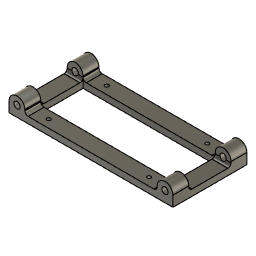
Pojezd - X v19 (Autodesk Fusion 360 design; units mm, degrees)
Autodesk Fusion 360 part; units mm, degrees
note: some values were not read from the file. Chosen so that the rebuilt part matches the saved one: which bodies a step acts on.
sketch "Sketch2" plane through (0, 0, 0) normal (0, 1, 0) x (1, 0, 0)
  circle A0 centre (0, -10) radius 3
  line L0 (147.5, -10) -> (147.5, 0)
  line L1 (147.5, 0) -> (-7.5, 0)
  line L2 (-7.5, 0) -> (-7.5, -10)
  arc A1 (-7.5, -10) -> (7.5, -10) centre (0, -10) ccw
  line L3 (7.5, -10) -> (7.5, -9)
  arc A2 (10.5, -6) -> (7.5, -9) centre (10.5, -9) ccw
  line L4 (70, 35) -> (70, -50) construction
  arc A3 (132.5, -10) -> (147.5, -10) centre (140, -10) ccw
  circle A4 centre (140, -10) radius 3
  line L5 (132.5, -10) -> (132.5, -9)
  arc A5 (132.5, -9) -> (129.5, -6) centre (129.5, -9) ccw
  line L6 (10.5, -6) -> (129.5, -6)
  dimension "d11" = 10
  dimension "d13" = 15
  dimension "d14" = 6
  dimension "d16" = 155
  dimension "d24" = 3
  dimension "d53" = 7.5
  dimension "d54" = 77.5
  dimension "d55" = 140
  dimension "d56" = 6
  dimension "d117" = 4
  constraint concentric A0 A1
  constraint vertical L0
  constraint horizontal L1
  constraint vertical L2
  constraint horizontal L6
  constraint vertical L3
  constraint tangent L3 A2
  constraint tangent A2 L6
  constraint perpendicular L4 L6
  constraint symmetric A0 L4 A4
  constraint symmetric A1 L4 A3
  constraint symmetric L2.end L4 L0.start
  constraint symmetric A1.end L4 A3.start
  constraint symmetric L3.end L4 L5.end
  constraint symmetric A2.start L4 A5.end
  constraint symmetric A2 L4 A5
  measures "d11" vertical distance of origin A0.centre
  measures "d13" diameter of A1
  measures "d14" diameter of A0
  measures "d16" distance of L0.end L1.end
  measures "d24" radius of A2
  measures "d53" distance of origin L1.end
  measures "d54" horizontal distance of L1.end L4.start
  measures "d55" distance of A0.centre A3.centre
  measures "d56" distance of L1 L6
  measures "d117" vertical distance of A0.centre A2.start
extrude "Extrude9" add sketch "Sketch2" along normal blind 70 makes body 1
sketch "Sketch6" plane through (0, 0, 0) normal (0, 0, 1) x (1, 0, 0)
  line L0 (0, -15) -> (0, 85) construction
  line L1 (147.5, 0) -> (147.5, 70)
  line L2 (147.5, 70) -> (-7.5, 70)
  line L3 (-7.5, 70) -> (-7.5, 0)
  line L4 (140, -10) -> (140, 85) construction
  line L5 (7.5, 55) -> (-7.5, 55)
  line L6 (-7.5, 15) -> (7.5, 15)
  line L7 (132.5, 55) -> (147.5, 55)
  line L8 (147.5, 15) -> (132.5, 15)
  line L9 (132.5, 15) -> (132.5, 55)
  line L10 (132.5, 55) -> (7.5, 55)
  line L11 (132.5, 15) -> (7.5, 15)
  line L12 (7.5, 55) -> (7.5, 15)
  circle A0 centre (22.5, 7.5) radius 1.75
  circle A1 centre (22.5, 62.5) radius 1.75
  line L13 (70, 85) -> (70, -15) construction
  circle A2 centre (117.5, 62.5) radius 1.75
  circle A3 centre (117.5, 7.5) radius 1.75
  line L14 (78, 1.6) -> (70.5, 1.6)
  line L15 (69, 13.5) -> (72, 10.5)
  line L16 (72, 10.5) -> (69, 7.6)
  line L17 (69, 7.6) -> (72, 4.6)
  line L18 (72, 4.6) -> (69, 1.6)
  line L19 (70.5, 13.5) -> (73.5, 10.5)
  line L20 (73.5, 10.5) -> (70.5, 7.6)
  line L21 (73.5, 4.6) -> (70.5, 1.6)
  line L22 (70.5, 7.6) -> (73.5, 4.6)
  line L23 (69, 13.5) -> (62.2186, 13.5)
  line L24 (62.2186, 13.5) -> (62.2186, 1.6)
  line L25 (69, 1.6) -> (62.2186, 1.6)
  line L26 (70.5, 13.5) -> (78, 13.5)
  line L27 (78, 13.5) -> (78, 1.6)
  line L28 (-7.5, 0) -> (147.5, 0)
  dimension "d59" = 7.5
  dimension "d60" = 155
  dimension "d61" = 70
  dimension "d62" = 70
  dimension "d63" = 140
  dimension "d64" = 155
  dimension "d66" = 7.5
  dimension "d67" = 15
  dimension "d68" = 15
  dimension "d69" = 15
  dimension "d70" = 15
  dimension "d71" = 15
  dimension "d73" = 15
  dimension "d77" = 15
  dimension "d78" = 15
  dimension "d99" = 3.5
  dimension "d100" = 30
  dimension "d101" = 7.5
  dimension "d102" = 3.5
  dimension "d103" = 30
  dimension "d104" = 7.5
  dimension "d105" = 77.5
  constraint vertical L0
  constraint horizontal L28
  constraint vertical L1
  constraint horizontal L2
  constraint vertical L3
  constraint vertical L4
  constraint perpendicular L7 L9
  constraint perpendicular L11 L12
  constraint symmetric A0 L13 A3
  constraint symmetric A1 L13 A2
  constraint horizontal L14
  constraint vertical L13
  constraint horizontal L23
  constraint vertical L24
  constraint horizontal L25
  constraint vertical L27
  constraint horizontal L26
  measures "d59" horizontal distance of origin L3.end
  measures "d60" distance of L3.end L1.start
  measures "d61" distance of L1.start L1.end
  measures "d62" vertical distance of origin L2.end
  measures "d63" distance of L0 L4
  measures "d64" horizontal distance of L6.start L8.start
  measures "d66" horizontal distance of origin L6.start
  measures "d67" distance of L6.start L6.end
  measures "d68" vertical distance of origin L6.start
  measures "d69" distance of L2.end L5.end
  measures "d70" distance of L5.start L5.end
  measures "d71" distance of L7.start L7.end
  measures "d73" distance of L8.start L8.end
  measures "d77" distance of L1.end L7.end
  measures "d78" distance of L1.start L8.start
  measures "d99" diameter of A0
  measures "d100" horizontal distance of L3.end A0.centre
  measures "d101" vertical distance of L3.end A0.centre
  measures "d102" diameter of A1
  measures "d103" horizontal distance of L2.end A1.centre
  measures "d104" vertical distance of L2.end A1.centre
  measures "d105" horizontal distance of L2.end L13.start
extrude "Extrude13" cut sketch "Sketch6" along normal blind 40 contours L1 L7 L8 L9 | L9 L10 L11 L12 | L3 L5 L6 L12 bodies 1 makes body 2 at (95.8333, 5, 0)
extrude "Extrude14" add sketch "Sketch6" along normal blind 6 contours L1 L7 L8 L9 | L3 L5 L6 L12 bodies 1 2
fillet "Fillet1" radius 3 1 edges at (140, 55, 6) on bodies 1
fillet "Fillet2" radius 3 1 edges at (140, 15, 6) on bodies 1
fillet "Fillet3" radius 3 1 edges at (0, 15, 6) on bodies 1
fillet "Fillet4" radius 3 1 edges at (0, 55, 6) on bodies 1
extrude "Extrude15" cut sketch "Sketch6" along normal blind 30 contours A0 | A1 | A2 | A3 bodies 1
extrude "Extrude10" [suppressed]
extrude "Extrude11" [suppressed]
extrude "Extrude12" [suppressed]
copy_body "Body->Comp1" [suppressed] in component "Úchytka"
named bodies: "Úchytka", "Tělo"
